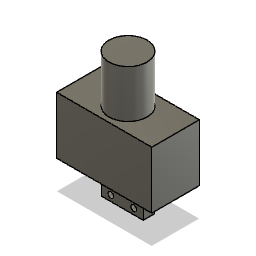
Base da garra v8 (Autodesk Fusion 360 design; units mm, degrees)
Autodesk Fusion 360 part; units mm, degrees
sketch "Sketch1" plane through (0, 0, 0) normal (0, 1, 0) x (1, 0, 0)
  line L0 (25, -12.5) -> (-25, -12.5)
  line L1 (-25, -12.5) -> (-25, 12.5)
  line L2 (-25, 12.5) -> (25, 12.5)
  line L3 (25, 12.5) -> (25, -12.5)
  line L4 (25, -12.5) -> (-25, 12.5) construction
  line L5 (-25, -12.5) -> (25, 12.5) construction
  dimension "d1" = 50
  dimension "d2" = 25
  constraint horizontal L0
  constraint perpendicular L0 L1
  constraint parallel L0 L2
  constraint parallel L1 L3
  constraint coincident L4 origin
  constraint coincident L5 origin
  measures "d1" distance of L1.end L2.end
  measures "d2" distance of L0.end L1.end
extrude "Extrude1" add sketch "Sketch1" along normal blind 30 makes body 1
sketch "Sketch2" plane through (0, 30, 0) normal (0, 1, 0) x (-1, 0, 0)
  line L0 (-25, -12.5) -> (25, -12.5)
  line L1 (25, -12.5) -> (25, 12.5)
  line L2 (25, 12.5) -> (-25, 12.5)
  line L3 (-25, 12.5) -> (-25, -12.5)
  circle A0 centre (0, 0) radius 10
  dimension "d5" = 20
  constraint coincident A0.centre origin
  measures "d5" diameter of A0
extrude "Extrude2" add sketch "Sketch2" along normal blind 25 contours A0 bodies 1
sketch "Sketch3" plane through (0, 0, 0) normal (0, -1, 0) x (1, 0, 0)
  line L0 (-25, -12.5) -> (25, -12.5)
  line L1 (25, -12.5) -> (25, 12.5)
  line L2 (25, 12.5) -> (-25, 12.5)
  line L3 (-25, 12.5) -> (-25, -12.5)
  line L4 (11, -3) -> (-11, -3)
  line L5 (-11, -3) -> (-11, 3)
  line L6 (-11, 3) -> (11, 3)
  line L7 (11, 3) -> (11, -3)
  line L8 (11, -3) -> (-11, 3) construction
  line L9 (-11, -3) -> (11, 3) construction
  dimension "d8" = 22
  dimension "d9" = 6
  constraint horizontal L4
  constraint perpendicular L4 L5
  constraint parallel L4 L6
  constraint parallel L5 L7
  constraint coincident L8 origin
  constraint coincident L9 origin
  measures "d8" distance of L5.end L6.end
  measures "d9" distance of L4.end L5.end
extrude "Extrude4" add sketch "Sketch3" along normal blind 10 contours L4 L5 L6 L7 bodies 1
sketch "Sketch4" plane through (0, 0, 3) normal (0, 0, 1) x (1, 0, 0)
  line L0 (11, 0) -> (-11, 0)
  line L1 (-11, 0) -> (-11, -10)
  line L2 (-11, -10) -> (11, -10)
  line L3 (11, -10) -> (11, 0)
  circle A0 centre (-6, -7) radius 1.5
  circle A1 centre (6, -7) radius 1.5
  dimension "d16" = 3
  dimension "d19" = 3
  measures "d16" diameter of A0
  measures "d19" diameter of A1
extrude "Extrude5" cut sketch "Sketch4" against normal blind 15 contours A0 | A1 bodies 1
extrude "Extrude3" add sketch "Sketch3" along normal blind 15 contours L4 L5 L6 L7 bodies 1
sketch "Sketch5" plane through (0, 0, 3) normal (0, 0, 1) x (1, 0, 0)
  line L0 (11, 0) -> (-11, 0)
  line L1 (-11, 0) -> (-11, -15)
  line L2 (-11, -15) -> (11, -15)
  line L3 (11, -15) -> (11, 0)
  circle A0 centre (-6, -12) radius 1.5
  circle A1 centre (6, -12) radius 1.5
  dimension "d26" = 3
  dimension "d27" = 3
  measures "d26" diameter of A0
  measures "d27" diameter of A1
extrude "Extrude6" cut sketch "Sketch5" against normal blind 21 contours A0 | A1 bodies 1
copy_body "Body->Comp2" bodies 1 removing the originals makes body 2 in component "Component"
component "Component" placed x (1, 0, 0) y (0, 1, 0) z (0, 0, 1) at (0, 0, 0)
